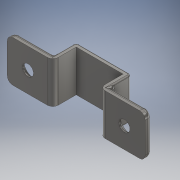
# Autodesk Inventor part: Latch Catch
Saved by Autodesk Inventor 2018 (Build 220112000, 112)
## iProperties
Created: 2018-10-16
Part Number: Latch Catch
Material: Steel
Document SubType Name: Modeling
Designer: P301319
Density: 7.85 g/cm^3
Appearance: Semi-Polished
Author: P301319
Autodesk Inventor part; units mm, degrees
ref_plane "YZ Plane" through (0, 0, 0) normal (1, 0, 0) x (0, 1, 0)
ref_plane "XZ Plane" through (0, 0, 0) normal (0, 1, 0) x (-1, 0, 0)
ref_plane "XY Plane" through (0, 0, 0) normal (0, 0, 1) x (1, 0, 0)
sketch "Sketch1" plane through (0, 0, 0) normal (0, 0, 1) x (1, 0, 0)
  line L0 (0, 0) -> (50, 0) construction
  line L1 (0, 0) -> (16.5, 0)
  line L2 (50, 0) -> (33.5, 0)
  line L3 (0, 0) -> (0, 2.5)
  line L4 (50, 0) -> (50, 2.5)
  line L5 (16.5, 0) -> (16.5, 8.5)
  line L6 (33.5, 0) -> (33.5, 8.5)
  line L7 (33.5, 8.5) -> (16.5, 8.5)
  line L8 (0, 2.5) -> (15, 2.5)
  line L9 (50, 2.5) -> (35, 2.5)
  line L10 (15, 2.5) -> (15, 10)
  line L11 (35, 2.5) -> (35, 10)
  line L12 (15, 10) -> (35, 10)
  dimension "d0" = 50
  dimension "d1" = 16.5
  dimension "d2" = 16.5
  dimension "d3" = 2.5
  dimension "d4" = 8.5
  dimension "d5" = 15
  dimension "d6" = 15
  dimension "d7" = 2.5
  dimension "d8" = 7.5
  dimension "d9" = 7.5
  constraints: 26 end point, 5 vertical, 4 horizontal, 2 point on line, 1 perpendicular
  measures "d0" distance of L0.start L0.end
  measures "d1" distance of L0.start L1.end
  measures "d2" distance of L0.end L2.end
  measures "d3" distance of L0.start L3.end
  measures "d4" distance of L1.end L5.end
  measures "d5" distance of L3.end L8.end
  measures "d6" distance of L4.end L9.end
  measures "d7" distance of L0.end L4.end
  measures "d8" distance of L8.end L10.end
  measures "d9" distance of L9.end L11.end
extrude "Extrusion1" add sketch "Sketch1" along normal blind 15
sketch "Sketch2" plane through (35, 2.5, 0) normal (0, 1, 0) x (1, 0, 0)
  line L0 (15, 0) -> (15, -15) projected
  line L1 (-35, 0) -> (-35, -15) projected
  point P0 (7.5, -7.5)
  point P1 (-27.5, -7.5)
  point P2 (15, -7.5)
  dimension "d12" = 7.5
  dimension "d13" = 7.5
  constraints: 2 horizontal alignment, 1 midpoint
  measures "d12" distance from line of L0 point (7.5, -7.5)
  measures "d13" distance from line of L1 point (-27.5, -7.5)
hole "Hole1" at (42.5, 2.5, 7.5) at (7.5, 2.5, 7.5) direction (0, -1, 0) diameter 4 end through all countersink diameter 8 countersink angle 90
fillet "Fillet5" radius 0.5 6 edges at (25, 10, 0) (15, 6.25, 0) (35, 6.25, 0) (15, 6.25, 15) (25, 10, 15) (35, 6.25, 15)
fillet "Fillet6" radius 1 6 edges at (15.1464, 9.8536, 14.8536) (15.1464, 9.8536, 0.1464) (15, 10, 7.5) (34.8536, 9.8536, 14.8536) (34.8536, 9.8536, 0.1464) (35, 10, 7.5)
fillet "Fillet7" radius 1.5 8 edges at (42.5, 2.5, 3.5) (7.5, 2.5, 3.5) (7.75, 2.5, 15) (0, 2.5, 7.5) (7.75, 2.5, 0) (42.25, 2.5, 0) (50, 2.5, 7.5) (42.25, 2.5, 15)
fillet "Fillet8" radius 2 10 edges at (33.5, 0, 7.5) (16.5, 0, 7.5) (0.4393, 2.0607, 0.4393) (0, 0.5, 0) (0, 0.5, 15) (0.4393, 2.0607, 14.5607) (50, 0.5, 0) (49.5607, 2.0607, 0.4393) (50, 0.5, 15) (49.5607, 2.0607, 14.5607)
fillet "Fillet9" radius 1.5 10 edges at (15, 2.4013, 14.0352) (15.1688, 1.6004, 14.8746) (15, 2.4013, 0.9648) (15.1688, 1.6004, 0.1254) (15, 2.5, 7.5) (35, 2.4013, 14.0352) (34.8312, 1.6004, 14.8746) (35, 2.4013, 0.9648) (34.8312, 1.6004, 0.1254) (35, 2.5, 7.5)
equation "\"d2\" = d1"
equation "\"d6\" = d5"
equation "\"d7\" = d3"
equation "\"d9\" = d8"
equation "\"d13\" = d12"
body "Solid1"
